Autodesk Fusion 360 part; units mm, degrees
note: some values were not read from the file. Set by a fixed rule: the direction of a hole.
(part 4 of 10)
  line L2847 (66.04, 10.795) -> (64.135, 10.795)
  line L2848 (64.135, 10.795) -> (54.61, 10.795)
  line L2849 (54.61, 10.795) -> (52.07, 10.795)
  line L2850 (67.31, 4.89) -> (67.31, 10.795)
  line L2851 (80.01, 4.89) -> (80.01, 10.795)
  line L2852 (4.635, 10.795) -> (15.24, 10.795)
  line L2853 (15.24, 10.795) -> (15.875, 10.795)
  line L2854 (15.875, 10.795) -> (25.4, 10.795)
  line L2855 (28.575, 10.795) -> (25.4, 10.795)
  line L2856 (28.575, 10.795) -> (38.1, 10.795)
  line L2857 (38.1, 10.795) -> (40.64, 10.795)
  line L2858 (40.64, 10.795) -> (41.275, 10.795)
  line L2859 (41.275, 10.795) -> (52.07, 10.795)
  line L2860 (41.275, 4.89) -> (41.275, 10.795)
  line L2861 (28.575, 4.89) -> (28.575, 10.795)
  line L2862 (15.875, 4.89) -> (15.875, 10.795)
  line L2863 (12.7, 16.51) -> (12.7, 11.43)
  line L2864 (12.7, 11.43) -> (25.4, 11.43)
  line L2865 (25.4, 11.43) -> (25.4, 10.795)
  line L2866 (25.4, 10.795) -> (25.4, 16.51)
  line L2867 (38.1, 16.51) -> (38.1, 10.795)
  line L2868 (64.77, 16.51) -> (64.77, 11.43)
  line L2869 (64.77, 11.43) -> (64.135, 10.795)
  line L2870 (76.2, 16.51) -> (76.2, 10.795)
  line L2871 (87.63, 16.51) -> (87.63, 11.43)
  line L2872 (87.63, 11.43) -> (88.265, 10.795)
  line L2873 (76.2, 76.2) -> (55.245, 76.2)
  line L2874 (55.245, 76.2) -> (54.165, 76.2)
  line L2875 (24.13, 76.835) -> (26.67, 76.835)
  line L2876 (32.8483, 78.7425) -> (32.8508, 78.74)
  line L2877 (50.8, 78.74) -> (32.8508, 78.74)
  line L2878 (26.67, 76.835) -> (28.5775, 78.7425)
  line L2879 (28.5775, 78.7425) -> (32.8483, 78.7425)
  line L2880 (53.34, 75.375) -> (50.8, 77.915)
  line L2881 (50.8, 77.915) -> (50.8, 78.74)
  line L2882 (53.34, 75.375) -> (54.165, 76.2)
  line L2883 (54.165, 76.2) -> (55.245, 76.2)
  line L2884 (88.265, 10.795) -> (95.44, 10.795)
  line L2885 (80.01, 4.89) -> (80.01, 4.445)
  line L2886 (53.34, 75.375) -> (53.34, 60.96)
  line L2887 (53.34, 60.96) -> (50.8, 58.42)
  line L2888 (36.534, 67.1383) -> (37.02, 67.235)
  line L2889 (37.918, 66.863) -> (38.1933, 66.451)
  line L2890 (36.122, 62.527) -> (35.8467, 62.939)
  line L2891 (36.534, 62.2517) -> (36.122, 62.527)
  line L2892 (38.1933, 62.939) -> (37.918, 62.527)
  line L2893 (38.29, 63.425) -> (38.1933, 62.939)
  line L2894 (37.506, 67.1383) -> (37.918, 66.863)
  line L2895 (35.75, 65.965) -> (35.8467, 66.451)
  line L2896 (36.122, 66.863) -> (36.534, 67.1383)
  line L2897 (35.8467, 66.451) -> (36.122, 66.863)
  line L2898 (35.75, 63.425) -> (35.75, 65.965)
  line L2899 (37.506, 62.2517) -> (37.02, 62.155)
  line L2900 (37.02, 62.155) -> (36.534, 62.2517)
  line L2901 (37.918, 62.527) -> (37.506, 62.2517)
  line L2902 (37.02, 67.235) -> (37.506, 67.1383)
  line L2903 (38.29, 65.965) -> (38.29, 63.425)
  line L2904 (38.1933, 66.451) -> (38.29, 65.965)
  line L2905 (35.8467, 62.939) -> (35.75, 63.425)
  line L2906 (2.25, 65.99) -> (2.3467, 66.476)
  line L2907 (3.034, 62.2767) -> (2.622, 62.552)
  line L2908 (4.79, 65.99) -> (4.79, 63.45)
  line L2909 (4.418, 62.552) -> (4.006, 62.2767)
  line L2910 (4.6933, 66.476) -> (4.79, 65.99)
  line L2911 (4.006, 67.1633) -> (4.418, 66.888)
  line L2912 (2.3467, 66.476) -> (2.622, 66.888)
  line L2913 (2.25, 63.45) -> (2.25, 65.99)
  line L2914 (2.3467, 62.964) -> (2.25, 63.45)
  line L2915 (4.79, 63.45) -> (4.6933, 62.964)
  line L2916 (2.622, 62.552) -> (2.3467, 62.964)
  line L2917 (4.006, 62.2767) -> (3.52, 62.18)
  line L2918 (2.622, 66.888) -> (3.034, 67.1633)
  line L2919 (4.6933, 62.964) -> (4.418, 62.552)
  line L2920 (3.034, 67.1633) -> (3.52, 67.26)
  line L2921 (3.52, 67.26) -> (4.006, 67.1633)
  line L2922 (4.418, 66.888) -> (4.6933, 66.476)
  line L2923 (3.52, 62.18) -> (3.034, 62.2767)
  line L2924 (64.208, 67.013) -> (64.4833, 66.601)
  line L2925 (63.31, 62.305) -> (62.824, 62.4017)
  line L2926 (62.412, 62.677) -> (62.1367, 63.089)
  line L2927 (64.4833, 63.089) -> (64.208, 62.677)
  line L2928 (63.796, 62.4017) -> (63.31, 62.305)
  line L2929 (64.208, 62.677) -> (63.796, 62.4017)
  line L2930 (64.58, 66.115) -> (64.58, 63.575)
  line L2931 (64.4833, 66.601) -> (64.58, 66.115)
  line L2932 (64.58, 63.575) -> (64.4833, 63.089)
  line L2933 (62.412, 67.013) -> (62.824, 67.2883)
  line L2934 (63.31, 67.385) -> (63.796, 67.2883)
  line L2935 (62.824, 67.2883) -> (63.31, 67.385)
  line L2936 (63.796, 67.2883) -> (64.208, 67.013)
  line L2937 (62.1367, 66.601) -> (62.412, 67.013)
  line L2938 (62.04, 66.115) -> (62.1367, 66.601)
  line L2939 (62.824, 62.4017) -> (62.412, 62.677)
  line L2940 (62.04, 63.575) -> (62.04, 66.115)
  line L2941 (62.1367, 63.089) -> (62.04, 63.575)
  line L2942 (96.81, 62.28) -> (96.324, 62.3767)
  line L2943 (95.912, 66.988) -> (96.324, 67.2633)
  line L2944 (97.708, 66.988) -> (97.9833, 66.576)
  line L2945 (96.81, 67.36) -> (97.296, 67.2633)
  line L2946 (95.912, 62.652) -> (95.6367, 63.064)
  line L2947 (95.6367, 63.064) -> (95.54, 63.55)
  line L2948 (97.296, 62.3767) -> (96.81, 62.28)
  line L2949 (96.324, 67.2633) -> (96.81, 67.36)
  line L2950 (95.6367, 66.576) -> (95.912, 66.988)
  line L2951 (95.54, 66.09) -> (95.6367, 66.576)
  line L2952 (97.296, 67.2633) -> (97.708, 66.988)
  line L2953 (97.9833, 66.576) -> (98.08, 66.09)
  line L2954 (98.08, 66.09) -> (98.08, 63.55)
  line L2955 (98.08, 63.55) -> (97.9833, 63.064)
  line L2956 (97.9833, 63.064) -> (97.708, 62.652)
  line L2957 (97.708, 62.652) -> (97.296, 62.3767)
  line L2958 (96.324, 62.3767) -> (95.912, 62.652)
  line L2959 (95.54, 63.55) -> (95.54, 66.09)
  line L2960 (8.0863, 54.243) -> (7.811, 53.831)
  line L2961 (3.475, 55.627) -> (3.887, 55.9023)
  line L2962 (6.913, 55.999) -> (7.399, 55.9023)
  line L2963 (8.0863, 55.215) -> (8.183, 54.729)
  line L2964 (3.1997, 54.243) -> (3.103, 54.729)
  line L2965 (4.373, 55.999) -> (6.913, 55.999)
  line L2966 (3.475, 53.831) -> (3.1997, 54.243)
  line L2967 (7.399, 55.9023) -> (7.811, 55.627)
  line L2968 (6.913, 53.459) -> (4.373, 53.459)
  line L2969 (4.373, 53.459) -> (3.887, 53.5557)
  line L2970 (8.183, 54.729) -> (8.0863, 54.243)
  line L2971 (3.103, 54.729) -> (3.1997, 55.215)
  line L2972 (3.887, 53.5557) -> (3.475, 53.831)
  line L2973 (7.811, 55.627) -> (8.0863, 55.215)
  line L2974 (7.811, 53.831) -> (7.399, 53.5557)
  line L2975 (3.887, 55.9023) -> (4.373, 55.999)
  line L2976 (3.1997, 55.215) -> (3.475, 55.627)
  line L2977 (7.399, 53.5557) -> (6.913, 53.459)
  line L2978 (3.887, 30.5557) -> (3.475, 30.831)
  line L2979 (4.373, 30.459) -> (3.887, 30.5557)
  line L2980 (6.913, 30.459) -> (4.373, 30.459)
  line L2981 (7.399, 32.9023) -> (7.811, 32.627)
  line L2982 (8.0863, 32.215) -> (8.183, 31.729)
  line L2983 (7.811, 30.831) -> (7.399, 30.5557)
  line L2984 (4.373, 32.999) -> (6.913, 32.999)
  line L2985 (3.887, 32.9023) -> (4.373, 32.999)
  line L2986 (3.475, 32.627) -> (3.887, 32.9023)
  line L2987 (3.475, 30.831) -> (3.1997, 31.243)
  line L2988 (3.1997, 32.215) -> (3.475, 32.627)
  line L2989 (6.913, 32.999) -> (7.399, 32.9023)
  line L2990 (3.103, 31.729) -> (3.1997, 32.215)
  line L2991 (3.1997, 31.243) -> (3.103, 31.729)
  line L2992 (8.0863, 31.243) -> (7.811, 30.831)
  line L2993 (7.399, 30.5557) -> (6.913, 30.459)
  line L2994 (7.811, 32.627) -> (8.0863, 32.215)
  line L2995 (8.183, 31.729) -> (8.0863, 31.243)
  line L2996 (20.099, 53.5557) -> (19.613, 53.459)
  line L2997 (15.803, 54.729) -> (15.8997, 55.215)
  line L2998 (19.613, 55.999) -> (20.099, 55.9023)
  line L2999 (19.613, 53.459) -> (17.073, 53.459)
  line L3000 (16.587, 53.5557) -> (16.175, 53.831)
  line L3001 (20.7863, 54.243) -> (20.511, 53.831)
  line L3002 (20.7863, 55.215) -> (20.883, 54.729)
  line L3003 (20.511, 55.627) -> (20.7863, 55.215)
  line L3004 (15.8997, 54.243) -> (15.803, 54.729)
  line L3005 (20.511, 53.831) -> (20.099, 53.5557)
  line L3006 (20.883, 54.729) -> (20.7863, 54.243)
  line L3007 (16.175, 53.831) -> (15.8997, 54.243)
  line L3008 (15.8997, 55.215) -> (16.175, 55.627)
  line L3009 (16.175, 55.627) -> (16.587, 55.9023)
  line L3010 (16.587, 55.9023) -> (17.073, 55.999)
  line L3011 (20.099, 55.9023) -> (20.511, 55.627)
  line L3012 (17.073, 53.459) -> (16.587, 53.5557)
  line L3013 (17.073, 55.999) -> (19.613, 55.999)
  line L3014 (15.803, 31.729) -> (15.8997, 32.215)
  line L3015 (17.073, 30.459) -> (16.587, 30.5557)
  line L3016 (20.099, 30.5557) -> (19.613, 30.459)
  line L3017 (15.8997, 31.243) -> (15.803, 31.729)
  line L3018 (16.175, 32.627) -> (16.587, 32.9023)
  line L3019 (16.175, 30.831) -> (15.8997, 31.243)
  line L3020 (16.587, 32.9023) -> (17.073, 32.999)
  line L3021 (20.511, 30.831) -> (20.099, 30.5557)
  line L3022 (20.7863, 31.243) -> (20.511, 30.831)
  line L3023 (19.613, 32.999) -> (20.099, 32.9023)
  line L3024 (20.099, 32.9023) -> (20.511, 32.627)
  line L3025 (17.073, 32.999) -> (19.613, 32.999)
  line L3026 (15.8997, 32.215) -> (16.175, 32.627)
  line L3027 (16.587, 30.5557) -> (16.175, 30.831)
  line L3028 (20.883, 31.729) -> (20.7863, 31.243)
  line L3029 (20.7863, 32.215) -> (20.883, 31.729)
  line L3030 (20.511, 32.627) -> (20.7863, 32.215)
  line L3031 (19.613, 30.459) -> (17.073, 30.459)
  line L3032 (29.287, 53.5557) -> (28.875, 53.831)
  line L3033 (33.583, 54.729) -> (33.4863, 54.243)
  line L3034 (32.313, 55.999) -> (32.799, 55.9023)
  line L3035 (33.211, 53.831) -> (32.799, 53.5557)
  line L3036 (33.4863, 54.243) -> (33.211, 53.831)
  line L3037 (28.875, 53.831) -> (28.5997, 54.243)
  line L3038 (32.799, 55.9023) -> (33.211, 55.627)
  line L3039 (28.5997, 55.215) -> (28.875, 55.627)
  line L3040 (29.773, 53.459) -> (29.287, 53.5557)
  line L3041 (28.875, 55.627) -> (29.287, 55.9023)
  line L3042 (28.503, 54.729) -> (28.5997, 55.215)
  line L3043 (33.4863, 55.215) -> (33.583, 54.729)
  line L3044 (32.799, 53.5557) -> (32.313, 53.459)
  line L3045 (28.5997, 54.243) -> (28.503, 54.729)
  line L3046 (29.287, 55.9023) -> (29.773, 55.999)
  line L3047 (33.211, 55.627) -> (33.4863, 55.215)
  line L3048 (32.313, 53.459) -> (29.773, 53.459)
  line L3049 (29.773, 55.999) -> (32.313, 55.999)
  line L3050 (29.773, 30.459) -> (29.287, 30.5557)
  line L3051 (32.313, 30.459) -> (29.773, 30.459)
  line L3052 (28.875, 30.831) -> (28.5997, 31.243)
  line L3053 (32.799, 30.5557) -> (32.313, 30.459)
  line L3054 (29.287, 30.5557) -> (28.875, 30.831)
  line L3055 (29.287, 32.9023) -> (29.773, 32.999)
  line L3056 (28.875, 32.627) -> (29.287, 32.9023)
  line L3057 (33.211, 32.627) -> (33.4863, 32.215)
  line L3058 (33.583, 31.729) -> (33.4863, 31.243)
  line L3059 (33.4863, 31.243) -> (33.211, 30.831)
  line L3060 (32.799, 32.9023) -> (33.211, 32.627)
  line L3061 (28.5997, 31.243) -> (28.503, 31.729)
  line L3062 (29.773, 32.999) -> (32.313, 32.999)
  line L3063 (28.5997, 32.215) -> (28.875, 32.627)
  line L3064 (33.211, 30.831) -> (32.799, 30.5557)
  line L3065 (33.4863, 32.215) -> (33.583, 31.729)
  line L3066 (32.313, 32.999) -> (32.799, 32.9023)
  line L3067 (28.503, 31.729) -> (28.5997, 32.215)
  line L3068 (41.575, 55.627) -> (41.987, 55.9023)
  line L3069 (45.499, 53.5557) -> (45.013, 53.459)
  line L3070 (41.987, 53.5557) -> (41.575, 53.831)
  line L3071 (45.499, 55.9023) -> (45.911, 55.627)
  line L3072 (41.575, 53.831) -> (41.2997, 54.243)
  line L3073 (46.283, 54.729) -> (46.1863, 54.243)
  line L3074 (41.2997, 54.243) -> (41.203, 54.729)
  line L3075 (45.911, 53.831) -> (45.499, 53.5557)
  line L3076 (45.013, 53.459) -> (42.473, 53.459)
  line L3077 (42.473, 55.999) -> (45.013, 55.999)
  line L3078 (45.013, 55.999) -> (45.499, 55.9023)
  line L3079 (41.203, 54.729) -> (41.2997, 55.215)
  line L3080 (46.1863, 55.215) -> (46.283, 54.729)
  line L3081 (45.911, 55.627) -> (46.1863, 55.215)
  line L3082 (41.987, 55.9023) -> (42.473, 55.999)
  line L3083 (41.2997, 55.215) -> (41.575, 55.627)
  line L3084 (42.473, 53.459) -> (41.987, 53.5557)
  line L3085 (46.1863, 54.243) -> (45.911, 53.831)
  line L3086 (45.911, 30.831) -> (45.499, 30.5557)
  line L3087 (46.1863, 32.215) -> (46.283, 31.729)
  line L3088 (45.013, 32.999) -> (45.499, 32.9023)
  line L3089 (45.911, 32.627) -> (46.1863, 32.215)
  line L3090 (46.1863, 31.243) -> (45.911, 30.831)
  line L3091 (45.499, 32.9023) -> (45.911, 32.627)
  line L3092 (45.013, 30.459) -> (42.473, 30.459)
  line L3093 (41.203, 31.729) -> (41.2997, 32.215)
  line L3094 (41.2997, 31.243) -> (41.203, 31.729)
  line L3095 (42.473, 30.459) -> (41.987, 30.5557)
  line L3096 (46.283, 31.729) -> (46.1863, 31.243)
  line L3097 (41.575, 32.627) -> (41.987, 32.9023)
  line L3098 (42.473, 32.999) -> (45.013, 32.999)
  line L3099 (41.987, 32.9023) -> (42.473, 32.999)
  line L3100 (41.575, 30.831) -> (41.2997, 31.243)
  line L3101 (41.2997, 32.215) -> (41.575, 32.627)
  line L3102 (41.987, 30.5557) -> (41.575, 30.831)
  line L3103 (45.499, 30.5557) -> (45.013, 30.459)
  line L3104 (58.348, 55.999) -> (58.834, 55.9023)
  line L3105 (55.808, 55.999) -> (58.348, 55.999)
  line L3106 (54.91, 55.627) -> (55.322, 55.9023)
  line L3107 (54.6347, 54.243) -> (54.538, 54.729)
  line L3108 (58.834, 53.5557) -> (58.348, 53.459)
  line L3109 (55.322, 53.5557) -> (54.91, 53.831)
  line L3110 (59.5213, 55.215) -> (59.618, 54.729)
  line L3111 (58.834, 55.9023) -> (59.246, 55.627)
  line L3112 (54.6347, 55.215) -> (54.91, 55.627)
  line L3113 (55.808, 53.459) -> (55.322, 53.5557)
  line L3114 (59.246, 53.831) -> (58.834, 53.5557)
  line L3115 (58.348, 53.459) -> (55.808, 53.459)
  line L3116 (59.618, 54.729) -> (59.5213, 54.243)
  line L3117 (59.5213, 54.243) -> (59.246, 53.831)
  line L3118 (59.246, 55.627) -> (59.5213, 55.215)
  line L3119 (54.538, 54.729) -> (54.6347, 55.215)
  line L3120 (55.322, 55.9023) -> (55.808, 55.999)
  line L3121 (54.91, 53.831) -> (54.6347, 54.243)
  line L3122 (54.6347, 31.243) -> (54.538, 31.729)
  line L3123 (59.618, 31.729) -> (59.5213, 31.243)
  line L3124 (59.246, 32.627) -> (59.5213, 32.215)
  line L3125 (54.6347, 32.215) -> (54.91, 32.627)
  line L3126 (59.5213, 32.215) -> (59.618, 31.729)
  line L3127 (59.5213, 31.243) -> (59.246, 30.831)
  line L3128 (54.91, 30.831) -> (54.6347, 31.243)
  line L3129 (55.808, 30.459) -> (55.322, 30.5557)
  line L3130 (58.348, 30.459) -> (55.808, 30.459)
  line L3131 (55.322, 32.9023) -> (55.808, 32.999)
  line L3132 (58.834, 32.9023) -> (59.246, 32.627)
  line L3133 (59.246, 30.831) -> (58.834, 30.5557)
  line L3134 (54.538, 31.729) -> (54.6347, 32.215)
  line L3135 (55.808, 32.999) -> (58.348, 32.999)
  line L3136 (54.91, 32.627) -> (55.322, 32.9023)
  line L3137 (58.348, 32.999) -> (58.834, 32.9023)
  line L3138 (58.834, 30.5557) -> (58.348, 30.459)
  line L3139 (55.322, 30.5557) -> (54.91, 30.831)
  line L3140 (72.318, 54.729) -> (72.2213, 54.243)
  line L3141 (68.022, 55.9023) -> (68.508, 55.999)
  line L3142 (71.534, 55.9023) -> (71.946, 55.627)
  line L3143 (67.3347, 55.215) -> (67.61, 55.627)
  line L3144 (71.946, 53.831) -> (71.534, 53.5557)
  line L3145 (68.508, 55.999) -> (71.048, 55.999)
  line L3146 (72.2213, 55.215) -> (72.318, 54.729)
  line L3147 (67.61, 55.627) -> (68.022, 55.9023)
  line L3148 (67.61, 53.831) -> (67.3347, 54.243)
  line L3149 (72.2213, 54.243) -> (71.946, 53.831)
  line L3150 (68.508, 53.459) -> (68.022, 53.5557)
  line L3151 (67.238, 54.729) -> (67.3347, 55.215)
  line L3152 (71.534, 53.5557) -> (71.048, 53.459)
  line L3153 (71.048, 55.999) -> (71.534, 55.9023)
  line L3154 (67.3347, 54.243) -> (67.238, 54.729)
  line L3155 (68.022, 53.5557) -> (67.61, 53.831)
  line L3156 (71.946, 55.627) -> (72.2213, 55.215)
  line L3157 (71.048, 53.459) -> (68.508, 53.459)
  line L3158 (68.508, 30.459) -> (68.022, 30.5557)
  line L3159 (68.022, 30.5557) -> (67.61, 30.831)
  line L3160 (71.946, 32.627) -> (72.2213, 32.215)
  line L3161 (71.946, 30.831) -> (71.534, 30.5557)
  line L3162 (72.2213, 31.243) -> (71.946, 30.831)
  line L3163 (71.048, 30.459) -> (68.508, 30.459)
  line L3164 (67.238, 31.729) -> (67.3347, 32.215)
  line L3165 (67.3347, 32.215) -> (67.61, 32.627)
  line L3166 (72.2213, 32.215) -> (72.318, 31.729)
  line L3167 (71.534, 32.9023) -> (71.946, 32.627)
  line L3168 (71.048, 32.999) -> (71.534, 32.9023)
  line L3169 (68.508, 32.999) -> (71.048, 32.999)
  line L3170 (67.61, 32.627) -> (68.022, 32.9023)
  line L3171 (67.61, 30.831) -> (67.3347, 31.243)
  line L3172 (68.022, 32.9023) -> (68.508, 32.999)
  line L3173 (67.3347, 31.243) -> (67.238, 31.729)
  line L3174 (72.318, 31.729) -> (72.2213, 31.243)
  line L3175 (71.534, 30.5557) -> (71.048, 30.459)
  line L3176 (84.9213, 54.243) -> (84.646, 53.831)
  line L3177 (80.722, 53.5557) -> (80.31, 53.831)
  line L3178 (80.0347, 54.243) -> (79.938, 54.729)
  line L3179 (81.208, 55.999) -> (83.748, 55.999)
  line L3180 (79.938, 54.729) -> (80.0347, 55.215)
  line L3181 (83.748, 53.459) -> (81.208, 53.459)
  line L3182 (84.9213, 55.215) -> (85.018, 54.729)
  line L3183 (81.208, 53.459) -> (80.722, 53.5557)
  line L3184 (83.748, 55.999) -> (84.234, 55.9023)
  line L3185 (84.646, 55.627) -> (84.9213, 55.215)
  line L3186 (80.31, 53.831) -> (80.0347, 54.243)
  line L3187 (84.646, 53.831) -> (84.234, 53.5557)
  line L3188 (84.234, 55.9023) -> (84.646, 55.627)
  line L3189 (85.018, 54.729) -> (84.9213, 54.243)
  line L3190 (80.722, 55.9023) -> (81.208, 55.999)
  line L3191 (84.234, 53.5557) -> (83.748, 53.459)
  line L3192 (80.31, 55.627) -> (80.722, 55.9023)
  line L3193 (80.0347, 55.215) -> (80.31, 55.627)
  line L3194 (84.9213, 32.215) -> (85.018, 31.729)
  line L3195 (83.748, 30.459) -> (81.208, 30.459)
  line L3196 (83.748, 32.999) -> (84.234, 32.9023)
  line L3197 (84.234, 32.9023) -> (84.646, 32.627)
  line L3198 (79.938, 31.729) -> (80.0347, 32.215)
  line L3199 (84.234, 30.5557) -> (83.748, 30.459)
  line L3200 (80.0347, 32.215) -> (80.31, 32.627)
  line L3201 (81.208, 32.999) -> (83.748, 32.999)
  line L3202 (81.208, 30.459) -> (80.722, 30.5557)
  line L3203 (84.646, 32.627) -> (84.9213, 32.215)
  line L3204 (80.31, 32.627) -> (80.722, 32.9023)
  line L3205 (85.018, 31.729) -> (84.9213, 31.243)
  line L3206 (80.0347, 31.243) -> (79.938, 31.729)
  line L3207 (84.9213, 31.243) -> (84.646, 30.831)
  line L3208 (80.31, 30.831) -> (80.0347, 31.243)
  line L3209 (80.722, 32.9023) -> (81.208, 32.999)
  line L3210 (80.722, 30.5557) -> (80.31, 30.831)
  line L3211 (84.646, 30.831) -> (84.234, 30.5557)
  line L3212 (95.813, 55.999) -> (96.299, 55.9023)
  line L3213 (93.273, 55.999) -> (95.813, 55.999)
  line L3214 (96.711, 55.627) -> (96.9863, 55.215)
  line L3215 (92.003, 54.729) -> (92.0997, 55.215)
  line L3216 (95.813, 53.459) -> (93.273, 53.459)
  line L3217 (92.375, 53.831) -> (92.0997, 54.243)
  line L3218 (92.375, 55.627) -> (92.787, 55.9023)
  line L3219 (96.711, 53.831) -> (96.299, 53.5557)
  line L3220 (96.9863, 55.215) -> (97.083, 54.729)
  line L3221 (96.299, 53.5557) -> (95.813, 53.459)
  line L3222 (92.0997, 54.243) -> (92.003, 54.729)
  line L3223 (92.0997, 55.215) -> (92.375, 55.627)
  line L3224 (93.273, 53.459) -> (92.787, 53.5557)
  line L3225 (96.299, 55.9023) -> (96.711, 55.627)
  line L3226 (96.9863, 54.243) -> (96.711, 53.831)
  line L3227 (97.083, 54.729) -> (96.9863, 54.243)
  line L3228 (92.787, 53.5557) -> (92.375, 53.831)
  line L3229 (92.787, 55.9023) -> (93.273, 55.999)
  line L3230 (93.273, 30.459) -> (92.787, 30.5557)
  line L3231 (96.299, 32.9023) -> (96.711, 32.627)
  line L3232 (95.813, 32.999) -> (96.299, 32.9023)
  line L3233 (96.9863, 32.215) -> (97.083, 31.729)
  line L3234 (96.9863, 31.243) -> (96.711, 30.831)
  line L3235 (96.711, 30.831) -> (96.299, 30.5557)
  line L3236 (92.375, 30.831) -> (92.0997, 31.243)
  line L3237 (97.083, 31.729) -> (96.9863, 31.243)
  line L3238 (92.787, 32.9023) -> (93.273, 32.999)
  line L3239 (92.375, 32.627) -> (92.787, 32.9023)
  line L3240 (93.273, 32.999) -> (95.813, 32.999)
  line L3241 (92.003, 31.729) -> (92.0997, 32.215)
  line L3242 (92.0997, 32.215) -> (92.375, 32.627)
  line L3243 (96.299, 30.5557) -> (95.813, 30.459)
  line L3244 (95.813, 30.459) -> (93.273, 30.459)
  line L3245 (92.0997, 31.243) -> (92.003, 31.729)
  line L3246 (92.787, 30.5557) -> (92.375, 30.831)
  line L3247 (96.711, 32.627) -> (96.9863, 32.215)
  line L3248 (48.26, 77.475) -> (48.6618, 77.3951)
  line L3249 (47.5175, 73.5825) -> (47.2899, 73.9232)
  line L3250 (47.21, 74.325) -> (47.21, 76.425)
  line L3251 (48.6618, 77.3951) -> (49.0025, 77.1675)
  line L3252 (49.0025, 73.5825) -> (48.6618, 73.3549)
  line L3253 (49.31, 74.325) -> (49.2301, 73.9232)
  line L3254 (47.21, 76.425) -> (47.2899, 76.8268)
  line L3255 (49.31, 76.425) -> (49.31, 74.325)
  line L3256 (49.0025, 77.1675) -> (49.2301, 76.8268)
  line L3257 (47.5175, 77.1675) -> (47.8582, 77.3951)
  line L3258 (47.8582, 73.3549) -> (47.5175, 73.5825)
  line L3259 (49.2301, 76.8268) -> (49.31, 76.425)
  line L3260 (49.2301, 73.9232) -> (49.0025, 73.5825)
  line L3261 (47.2899, 76.8268) -> (47.5175, 77.1675)
  line L3262 (47.8582, 77.3951) -> (48.26, 77.475)
  line L3263 (47.2899, 73.9232) -> (47.21, 74.325)
  line L3264 (48.26, 73.275) -> (47.8582, 73.3549)
  line L3265 (48.6618, 73.3549) -> (48.26, 73.275)
  line L3266 (52.3699, 76.8268) -> (52.5975, 77.1675)
  line L3267 (54.3101, 76.8268) -> (54.39, 76.425)
  line L3268 (52.5975, 73.5825) -> (52.3699, 73.9232)
  line L3269 (52.29, 74.325) -> (52.29, 76.425)
  line L3270 (52.3699, 73.9232) -> (52.29, 74.325)
  line L3271 (52.9382, 77.3951) -> (53.34, 77.475)
  line L3272 (53.7418, 77.3951) -> (54.0825, 77.1675)
  line L3273 (54.3101, 73.9232) -> (54.0825, 73.5825)
  line L3274 (54.0825, 77.1675) -> (54.3101, 76.8268)
  line L3275 (52.29, 76.425) -> (52.3699, 76.8268)
  line L3276 (52.5975, 77.1675) -> (52.9382, 77.3951)
  line L3277 (53.7418, 73.3549) -> (53.34, 73.275)
  line L3278 (53.34, 73.275) -> (52.9382, 73.3549)
  line L3279 (54.39, 76.425) -> (54.39, 74.325)
  line L3280 (54.39, 74.325) -> (54.3101, 73.9232)
  line L3281 (53.34, 77.475) -> (53.7418, 77.3951)
  line L3282 (54.0825, 73.5825) -> (53.7418, 73.3549)
  line L3283 (52.9382, 73.3549) -> (52.5975, 73.5825)
  line L3284 (2.535, 10.795) -> (2.6149, 11.1968)
  line L3285 (6.4275, 10.0525) -> (6.0868, 9.8249)
  line L3286 (6.6551, 11.1968) -> (6.735, 10.795)
  line L3287 (5.685, 9.745) -> (3.585, 9.745)
  line L3288 (3.1832, 11.7651) -> (3.585, 11.845)
  line L3289 (3.1832, 9.8249) -> (2.8425, 10.0525)
  line L3290 (6.4275, 11.5375) -> (6.6551, 11.1968)
  line L3291 (6.6551, 10.3932) -> (6.4275, 10.0525)
  line L3292 (2.6149, 11.1968) -> (2.8425, 11.5375)
  line L3293 (6.735, 10.795) -> (6.6551, 10.3932)
  line L3294 (3.585, 9.745) -> (3.1832, 9.8249)
  line L3295 (2.6149, 10.3932) -> (2.535, 10.795)
  line L3296 (2.8425, 11.5375) -> (3.1832, 11.7651)
  line L3297 (2.8425, 10.0525) -> (2.6149, 10.3932)
  line L3298 (6.0868, 9.8249) -> (5.685, 9.745)
  line L3299 (5.685, 11.845) -> (6.0868, 11.7651)
  line L3300 (6.0868, 11.7651) -> (6.4275, 11.5375)
  line L3301 (3.585, 11.845) -> (5.685, 11.845)
  line L3302 (6.6551, 15.4732) -> (6.4275, 15.1325)
  line L3303 (5.685, 14.825) -> (3.585, 14.825)
  line L3304 (6.0868, 14.9049) -> (5.685, 14.825)
  line L3305 (6.6551, 16.2768) -> (6.735, 15.875)
  line L3306 (3.585, 16.925) -> (5.685, 16.925)
  line L3307 (2.535, 15.875) -> (2.6149, 16.2768)
  line L3308 (2.8425, 16.6175) -> (3.1832, 16.8451)
  line L3309 (2.6149, 15.4732) -> (2.535, 15.875)
  line L3310 (2.8425, 15.1325) -> (2.6149, 15.4732)
  line L3311 (6.735, 15.875) -> (6.6551, 15.4732)
  line L3312 (3.1832, 16.8451) -> (3.585, 16.925)
  line L3313 (6.4275, 16.6175) -> (6.6551, 16.2768)
  line L3314 (6.0868, 16.8451) -> (6.4275, 16.6175)
  line L3315 (3.1832, 14.9049) -> (2.8425, 15.1325)
  line L3316 (2.6149, 16.2768) -> (2.8425, 16.6175)
  line L3317 (3.585, 14.825) -> (3.1832, 14.9049)
  line L3318 (6.4275, 15.1325) -> (6.0868, 14.9049)
  line L3319 (5.685, 16.925) -> (6.0868, 16.8451)
  line L3320 (16.6175, 3.0975) -> (16.2768, 2.8699)
  line L3321 (16.6175, 6.6825) -> (16.8451, 6.3418)
  line L3322 (16.2768, 6.9101) -> (16.6175, 6.6825)
  line L3323 (15.875, 2.79) -> (15.4732, 2.8699)
  line L3324 (14.9049, 6.3418) -> (15.1325, 6.6825)
  line L3325 (16.925, 3.84) -> (16.8451, 3.4382)
  line L3326 (14.825, 5.94) -> (14.9049, 6.3418)
  line L3327 (15.1325, 3.0975) -> (14.9049, 3.4382)
  line L3328 (15.4732, 2.8699) -> (15.1325, 3.0975)
  line L3329 (14.9049, 3.4382) -> (14.825, 3.84)
  line L3330 (14.825, 3.84) -> (14.825, 5.94)
  line L3331 (16.925, 5.94) -> (16.925, 3.84)
  line L3332 (15.875, 6.99) -> (16.2768, 6.9101)
  line L3333 (16.2768, 2.8699) -> (15.875, 2.79)
  line L3334 (15.1325, 6.6825) -> (15.4732, 6.9101)
  line L3335 (16.8451, 3.4382) -> (16.6175, 3.0975)
  line L3336 (15.4732, 6.9101) -> (15.875, 6.99)
  line L3337 (16.8451, 6.3418) -> (16.925, 5.94)
  line L3338 (19.905, 5.94) -> (19.9849, 6.3418)
  line L3339 (21.6975, 6.6825) -> (21.9251, 6.3418)
  line L3340 (21.9251, 3.4382) -> (21.6975, 3.0975)
  line L3341 (22.005, 5.94) -> (22.005, 3.84)
  line L3342 (20.955, 6.99) -> (21.3568, 6.9101)
  line L3343 (20.2125, 6.6825) -> (20.5532, 6.9101)
  line L3344 (19.9849, 3.4382) -> (19.905, 3.84)
  line L3345 (20.955, 2.79) -> (20.5532, 2.8699)
  line L3346 (20.2125, 3.0975) -> (19.9849, 3.4382)
  line L3347 (19.9849, 6.3418) -> (20.2125, 6.6825)
  line L3348 (21.9251, 6.3418) -> (22.005, 5.94)
  line L3349 (20.5532, 2.8699) -> (20.2125, 3.0975)
  line L3350 (21.3568, 2.8699) -> (20.955, 2.79)
  line L3351 (21.3568, 6.9101) -> (21.6975, 6.6825)
  line L3352 (22.005, 3.84) -> (21.9251, 3.4382)
  line L3353 (21.6975, 3.0975) -> (21.3568, 2.8699)
  line L3354 (19.905, 3.84) -> (19.905, 5.94)
  line L3355 (20.5532, 6.9101) -> (20.955, 6.99)
  line L3356 (28.9768, 2.8699) -> (28.575, 2.79)
  line L3357 (27.525, 3.84) -> (27.525, 5.94)
  line L3358 (29.3175, 6.6825) -> (29.5451, 6.3418)
  line L3359 (27.6049, 6.3418) -> (27.8325, 6.6825)
  line L3360 (27.8325, 6.6825) -> (28.1732, 6.9101)
  line L3361 (29.625, 3.84) -> (29.5451, 3.4382)
  line L3362 (29.5451, 6.3418) -> (29.625, 5.94)
  line L3363 (29.625, 5.94) -> (29.625, 3.84)
  line L3364 (27.525, 5.94) -> (27.6049, 6.3418)
  line L3365 (28.9768, 6.9101) -> (29.3175, 6.6825)
  line L3366 (28.575, 2.79) -> (28.1732, 2.8699)
  line L3367 (29.3175, 3.0975) -> (28.9768, 2.8699)
  line L3368 (28.1732, 6.9101) -> (28.575, 6.99)
  line L3369 (28.1732, 2.8699) -> (27.8325, 3.0975)
  line L3370 (29.5451, 3.4382) -> (29.3175, 3.0975)
  line L3371 (27.8325, 3.0975) -> (27.6049, 3.4382)
  line L3372 (28.575, 6.99) -> (28.9768, 6.9101)
  line L3373 (27.6049, 3.4382) -> (27.525, 3.84)
  line L3374 (34.0568, 6.9101) -> (34.3975, 6.6825)
  line L3375 (34.6251, 3.4382) -> (34.3975, 3.0975)
  line L3376 (34.705, 5.94) -> (34.705, 3.84)
  line L3377 (34.705, 3.84) -> (34.6251, 3.4382)
  line L3378 (34.3975, 3.0975) -> (34.0568, 2.8699)
  line L3379 (34.6251, 6.3418) -> (34.705, 5.94)
  line L3380 (32.9125, 3.0975) -> (32.6849, 3.4382)
  line L3381 (32.6849, 3.4382) -> (32.605, 3.84)
  line L3382 (33.2532, 2.8699) -> (32.9125, 3.0975)
  line L3383 (34.0568, 2.8699) -> (33.655, 2.79)
  line L3384 (34.3975, 6.6825) -> (34.6251, 6.3418)
  line L3385 (32.605, 5.94) -> (32.6849, 6.3418)
  line L3386 (33.2532, 6.9101) -> (33.655, 6.99)
  line L3387 (33.655, 2.79) -> (33.2532, 2.8699)
  line L3388 (32.6849, 6.3418) -> (32.9125, 6.6825)
  line L3389 (33.655, 6.99) -> (34.0568, 6.9101)
  line L3390 (32.605, 3.84) -> (32.605, 5.94)
  line L3391 (32.9125, 6.6825) -> (33.2532, 6.9101)
  line L3392 (41.6768, 2.8699) -> (41.275, 2.79)
  line L3393 (40.5325, 6.6825) -> (40.8732, 6.9101)
  line L3394 (42.2451, 3.4382) -> (42.0175, 3.0975)
  line L3395 (40.225, 5.94) -> (40.3049, 6.3418)
  line L3396 (42.325, 5.94) -> (42.325, 3.84)
  line L3397 (41.6768, 6.9101) -> (42.0175, 6.6825)
  line L3398 (40.8732, 2.8699) -> (40.5325, 3.0975)
  line L3399 (40.5325, 3.0975) -> (40.3049, 3.4382)
  line L3400 (40.8732, 6.9101) -> (41.275, 6.99)
  line L3401 (41.275, 6.99) -> (41.6768, 6.9101)
  line L3402 (40.225, 3.84) -> (40.225, 5.94)
  line L3403 (42.325, 3.84) -> (42.2451, 3.4382)
  line L3404 (40.3049, 6.3418) -> (40.5325, 6.6825)
  line L3405 (40.3049, 3.4382) -> (40.225, 3.84)
  line L3406 (42.0175, 3.0975) -> (41.6768, 2.8699)
  line L3407 (42.0175, 6.6825) -> (42.2451, 6.3418)
  line L3408 (41.275, 2.79) -> (40.8732, 2.8699)
  line L3409 (42.2451, 6.3418) -> (42.325, 5.94)
  line L3410 (45.9532, 2.8699) -> (45.6125, 3.0975)
  line L3411 (46.355, 2.79) -> (45.9532, 2.8699)
  line L3412 (45.3849, 3.4382) -> (45.305, 3.84)
  line L3413 (45.9532, 6.9101) -> (46.355, 6.99)
  line L3414 (45.305, 5.94) -> (45.3849, 6.3418)
  line L3415 (46.355, 6.99) -> (46.7568, 6.9101)
  line L3416 (47.405, 3.84) -> (47.3251, 3.4382)
  line L3417 (47.3251, 3.4382) -> (47.0975, 3.0975)
  line L3418 (47.405, 5.94) -> (47.405, 3.84)
  line L3419 (46.7568, 2.8699) -> (46.355, 2.79)
  line L3420 (45.3849, 6.3418) -> (45.6125, 6.6825)
  line L3421 (45.305, 3.84) -> (45.305, 5.94)
  line L3422 (47.3251, 6.3418) -> (47.405, 5.94)
  line L3423 (47.0975, 6.6825) -> (47.3251, 6.3418)
  line L3424 (45.6125, 3.0975) -> (45.3849, 3.4382)
  line L3425 (46.7568, 6.9101) -> (47.0975, 6.6825)
  line L3426 (45.6125, 6.6825) -> (45.9532, 6.9101)
  line L3427 (47.0975, 3.0975) -> (46.7568, 2.8699)
  line L3428 (55.66, 3.84) -> (55.5801, 3.4382)
  line L3429 (54.61, 6.99) -> (55.0118, 6.9101)
  line L3430 (55.0118, 2.8699) -> (54.61, 2.79)
  line L3431 (55.3525, 3.0975) -> (55.0118, 2.8699)
  line L3432 (55.66, 5.94) -> (55.66, 3.84)
  line L3433 (53.56, 3.84) -> (53.56, 5.94)
  line L3434 (53.8675, 3.0975) -> (53.6399, 3.4382)
  line L3435 (55.5801, 3.4382) -> (55.3525, 3.0975)
  line L3436 (54.2082, 2.8699) -> (53.8675, 3.0975)
  line L3437 (55.5801, 6.3418) -> (55.66, 5.94)
  line L3438 (53.6399, 3.4382) -> (53.56, 3.84)
  line L3439 (54.2082, 6.9101) -> (54.61, 6.99)
  line L3440 (53.8675, 6.6825) -> (54.2082, 6.9101)
  line L3441 (55.0118, 6.9101) -> (55.3525, 6.6825)
  line L3442 (55.3525, 6.6825) -> (55.5801, 6.3418)
  line L3443 (53.6399, 6.3418) -> (53.8675, 6.6825)
  line L3444 (54.61, 2.79) -> (54.2082, 2.8699)
  line L3445 (53.56, 5.94) -> (53.6399, 6.3418)
  line L3446 (58.7199, 3.4382) -> (58.64, 3.84)
  line L3447 (60.0918, 6.9101) -> (60.4325, 6.6825)
  line L3448 (59.2882, 6.9101) -> (59.69, 6.99)
  line L3449 (58.7199, 6.3418) -> (58.9475, 6.6825)
  line L3450 (60.0918, 2.8699) -> (59.69, 2.79)
  line L3451 (58.64, 3.84) -> (58.64, 5.94)
  line L3452 (59.69, 6.99) -> (60.0918, 6.9101)
  line L3453 (58.9475, 3.0975) -> (58.7199, 3.4382)
  line L3454 (60.4325, 3.0975) -> (60.0918, 2.8699)
  line L3455 (60.6601, 3.4382) -> (60.4325, 3.0975)
  line L3456 (58.64, 5.94) -> (58.7199, 6.3418)
  line L3457 (59.2882, 2.8699) -> (58.9475, 3.0975)
  line L3458 (60.4325, 6.6825) -> (60.6601, 6.3418)
  line L3459 (60.6601, 6.3418) -> (60.74, 5.94)
  line L3460 (60.74, 5.94) -> (60.74, 3.84)
  line L3461 (58.9475, 6.6825) -> (59.2882, 6.9101)
  line L3462 (60.74, 3.84) -> (60.6601, 3.4382)
  line L3463 (59.69, 2.79) -> (59.2882, 2.8699)
  line L3464 (68.0525, 6.6825) -> (68.2801, 6.3418)
  line L3465 (66.3399, 3.4382) -> (66.26, 3.84)
  line L3466 (66.26, 5.94) -> (66.3399, 6.3418)
  line L3467 (66.3399, 6.3418) -> (66.5675, 6.6825)
  line L3468 (67.7118, 2.8699) -> (67.31, 2.79)
  line L3469 (66.5675, 3.0975) -> (66.3399, 3.4382)
  line L3470 (67.31, 2.79) -> (66.9082, 2.8699)
  line L3471 (66.26, 3.84) -> (66.26, 5.94)
  line L3472 (67.31, 6.99) -> (67.7118, 6.9101)
  line L3473 (66.9082, 2.8699) -> (66.5675, 3.0975)
  line L3474 (66.5675, 6.6825) -> (66.9082, 6.9101)
  line L3475 (66.9082, 6.9101) -> (67.31, 6.99)
  line L3476 (68.36, 3.84) -> (68.2801, 3.4382)
  line L3477 (68.2801, 3.4382) -> (68.0525, 3.0975)
  line L3478 (68.2801, 6.3418) -> (68.36, 5.94)
  line L3479 (67.7118, 6.9101) -> (68.0525, 6.6825)
  line L3480 (68.0525, 3.0975) -> (67.7118, 2.8699)
  line L3481 (68.36, 5.94) -> (68.36, 3.84)
  line L3482 (73.3601, 3.4382) -> (73.1325, 3.0975)
  line L3483 (71.34, 5.94) -> (71.4199, 6.3418)
  line L3484 (73.44, 3.84) -> (73.3601, 3.4382)
  line L3485 (72.7918, 6.9101) -> (73.1325, 6.6825)
  line L3486 (71.9882, 6.9101) -> (72.39, 6.99)
  line L3487 (73.1325, 6.6825) -> (73.3601, 6.3418)
  line L3488 (71.6475, 6.6825) -> (71.9882, 6.9101)
  line L3489 (71.34, 3.84) -> (71.34, 5.94)
  line L3490 (71.9882, 2.8699) -> (71.6475, 3.0975)
  line L3491 (72.39, 2.79) -> (71.9882, 2.8699)
  line L3492 (71.4199, 3.4382) -> (71.34, 3.84)
  line L3493 (72.7918, 2.8699) -> (72.39, 2.79)
  line L3494 (73.44, 5.94) -> (73.44, 3.84)
  line L3495 (73.1325, 3.0975) -> (72.7918, 2.8699)
  line L3496 (72.39, 6.99) -> (72.7918, 6.9101)
  line L3497 (71.4199, 6.3418) -> (71.6475, 6.6825)
  line L3498 (71.6475, 3.0975) -> (71.4199, 3.4382)
  line L3499 (73.3601, 6.3418) -> (73.44, 5.94)
  line L3500 (81.06, 5.94) -> (81.06, 3.84)
  line L3501 (80.9801, 3.4382) -> (80.7525, 3.0975)
  line L3502 (79.2675, 3.0975) -> (79.0399, 3.4382)
  line L3503 (78.96, 3.84) -> (78.96, 5.94)
  line L3504 (79.6082, 6.9101) -> (80.01, 6.99)
  line L3505 (80.7525, 6.6825) -> (80.9801, 6.3418)
  line L3506 (80.4118, 2.8699) -> (80.01, 2.79)
  line L3507 (80.9801, 6.3418) -> (81.06, 5.94)
  line L3508 (78.96, 5.94) -> (79.0399, 6.3418)
  line L3509 (80.01, 6.99) -> (80.4118, 6.9101)
  line L3510 (79.0399, 3.4382) -> (78.96, 3.84)
  line L3511 (79.0399, 6.3418) -> (79.2675, 6.6825)
  line L3512 (80.01, 2.79) -> (79.6082, 2.8699)
  line L3513 (80.7525, 3.0975) -> (80.4118, 2.8699)
  line L3514 (81.06, 3.84) -> (80.9801, 3.4382)
  line L3515 (79.6082, 2.8699) -> (79.2675, 3.0975)
  line L3516 (80.4118, 6.9101) -> (80.7525, 6.6825)
  line L3517 (79.2675, 6.6825) -> (79.6082, 6.9101)
  line L3518 (84.3475, 3.0975) -> (84.1199, 3.4382)
  line L3519 (85.4918, 6.9101) -> (85.8325, 6.6825)
  line L3520 (85.09, 2.79) -> (84.6882, 2.8699)
  line L3521 (85.8325, 6.6825) -> (86.0601, 6.3418)
  line L3522 (84.04, 3.84) -> (84.04, 5.94)
  line L3523 (84.6882, 2.8699) -> (84.3475, 3.0975)
  line L3524 (86.14, 3.84) -> (86.0601, 3.4382)
  line L3525 (84.1199, 3.4382) -> (84.04, 3.84)
  line L3526 (86.0601, 6.3418) -> (86.14, 5.94)
  line L3527 (85.4918, 2.8699) -> (85.09, 2.79)
  line L3528 (84.1199, 6.3418) -> (84.3475, 6.6825)
  line L3529 (85.8325, 3.0975) -> (85.4918, 2.8699)
  line L3530 (84.04, 5.94) -> (84.1199, 6.3418)
  line L3531 (84.3475, 6.6825) -> (84.6882, 6.9101)
  line L3532 (85.09, 6.99) -> (85.4918, 6.9101)
  line L3533 (84.6882, 6.9101) -> (85.09, 6.99)
  line L3534 (86.14, 5.94) -> (86.14, 3.84)
  line L3535 (86.0601, 3.4382) -> (85.8325, 3.0975)
  line L3536 (96.49, 9.745) -> (94.39, 9.745)
  line L3537 (93.6475, 11.5375) -> (93.9882, 11.7651)
  line L3538 (97.4601, 10.3932) -> (97.2325, 10.0525)
  line L3539 (97.2325, 11.5375) -> (97.4601, 11.1968)
  line L3540 (97.4601, 11.1968) -> (97.54, 10.795)
  line L3541 (93.6475, 10.0525) -> (93.4199, 10.3932)
  line L3542 (93.34, 10.795) -> (93.4199, 11.1968)
  line L3543 (94.39, 9.745) -> (93.9882, 9.8249)
  line L3544 (96.49, 11.845) -> (96.8918, 11.7651)
  line L3545 (97.2325, 10.0525) -> (96.8918, 9.8249)
  line L3546 (93.9882, 9.8249) -> (93.6475, 10.0525)
  line L3547 (96.8918, 9.8249) -> (96.49, 9.745)
  line L3548 (93.4199, 10.3932) -> (93.34, 10.795)
  line L3549 (94.39, 11.845) -> (96.49, 11.845)
  line L3550 (96.8918, 11.7651) -> (97.2325, 11.5375)
  line L3551 (97.54, 10.795) -> (97.4601, 10.3932)
  line L3552 (93.4199, 11.1968) -> (93.6475, 11.5375)
  line L3553 (93.9882, 11.7651) -> (94.39, 11.845)
  line L3554 (93.34, 15.875) -> (93.4199, 16.2768)
  line L3555 (96.8918, 14.9049) -> (96.49, 14.825)
  line L3556 (93.9882, 14.9049) -> (93.6475, 15.1325)
  line L3557 (96.49, 14.825) -> (94.39, 14.825)
  line L3558 (97.4601, 15.4732) -> (97.2325, 15.1325)
  line L3559 (93.6475, 15.1325) -> (93.4199, 15.4732)
  line L3560 (93.4199, 15.4732) -> (93.34, 15.875)
  line L3561 (97.2325, 16.6175) -> (97.4601, 16.2768)
  line L3562 (94.39, 14.825) -> (93.9882, 14.9049)
  line L3563 (94.39, 16.925) -> (96.49, 16.925)
  line L3564 (96.49, 16.925) -> (96.8918, 16.8451)
  line L3565 (93.4199, 16.2768) -> (93.6475, 16.6175)
  line L3566 (93.6475, 16.6175) -> (93.9882, 16.8451)
  line L3567 (93.9882, 16.8451) -> (94.39, 16.925)
  line L3568 (97.54, 15.875) -> (97.4601, 15.4732)
  line L3569 (97.2325, 15.1325) -> (96.8918, 14.9049)
  line L3570 (96.8918, 16.8451) -> (97.2325, 16.6175)
  line L3571 (97.4601, 16.2768) -> (97.54, 15.875)
  line L3572 (21.2598, 76.1746) -> (20.9296, 76.5048)
  line L3573 (22.2504, 76.5048) -> (21.9202, 76.1746)
  line L3574 (21.9202, 77.4954) -> (22.2504, 77.1652)
  line L3575 (21.2598, 77.4954) -> (21.9202, 77.4954)
  line L3576 (21.9202, 76.1746) -> (21.2598, 76.1746)
  line L3577 (22.2504, 77.1652) -> (22.2504, 76.5048)
  line L3578 (20.9296, 77.1652) -> (21.2598, 77.4954)
  line L3579 (20.9296, 76.5048) -> (20.9296, 77.1652)
  line L3580 (24.4602, 76.1746) -> (23.7998, 76.1746)
  line L3581 (23.4696, 76.5048) -> (23.4696, 77.1652)
  line L3582 (23.7998, 76.1746) -> (23.4696, 76.5048)
  line L3583 (24.7904, 76.5048) -> (24.4602, 76.1746)
  line L3584 (23.4696, 77.1652) -> (23.7998, 77.4954)
  line L3585 (23.7998, 77.4954) -> (24.4602, 77.4954)
  line L3586 (24.7904, 77.1652) -> (24.7904, 76.5048)
  line L3587 (24.4602, 77.4954) -> (24.7904, 77.1652)
  line L3588 (79.0702, 76.8604) -> (79.4004, 76.5302)
  line L3589 (78.4098, 75.5396) -> (78.0796, 75.8698)
  line L3590 (78.0796, 75.8698) -> (78.0796, 76.5302)
  line L3591 (78.0796, 76.5302) -> (78.4098, 76.8604)
  line L3592 (79.4004, 75.8698) -> (79.0702, 75.5396)
  line L3593 (79.0702, 75.5396) -> (78.4098, 75.5396)
  line L3594 (78.4098, 76.8604) -> (79.0702, 76.8604)
  line L3595 (79.4004, 76.5302) -> (79.4004, 75.8698)
  line L3596 (76.8604, 75.8698) -> (76.5302, 75.5396)
  line L3597 (76.5302, 75.5396) -> (75.8698, 75.5396)
  line L3598 (75.5396, 75.8698) -> (75.5396, 76.5302)
  line L3599 (75.8698, 76.8604) -> (76.5302, 76.8604)
  line L3600 (76.5302, 76.8604) -> (76.8604, 76.5302)
  line L3601 (75.8698, 75.5396) -> (75.5396, 75.8698)
  line L3602 (75.5396, 76.5302) -> (75.8698, 76.8604)
  line L3603 (76.8604, 76.5302) -> (76.8604, 75.8698)
  line L3604 (10.8204, 16.1798) -> (10.4902, 15.8496)
  line L3605 (9.4996, 16.8402) -> (9.8298, 17.1704)
  line L3606 (10.4902, 17.1704) -> (10.8204, 16.8402)
  line L3607 (10.4902, 15.8496) -> (9.8298, 15.8496)
  line L3608 (10.8204, 16.8402) -> (10.8204, 16.1798)
  line L3609 (9.4996, 16.1798) -> (9.4996, 16.8402)
  line L3610 (9.8298, 17.1704) -> (10.4902, 17.1704)
  line L3611 (9.8298, 15.8496) -> (9.4996, 16.1798)
  line L3612 (12.3698, 17.1704) -> (13.0302, 17.1704)
  line L3613 (13.3604, 16.8402) -> (13.3604, 16.1798)
  line L3614 (13.0302, 15.8496) -> (12.3698, 15.8496)
  line L3615 (12.0396, 16.1798) -> (12.0396, 16.8402)
  line L3616 (12.3698, 15.8496) -> (12.0396, 16.1798)
  line L3617 (13.3604, 16.1798) -> (13.0302, 15.8496)
  line L3618 (13.0302, 17.1704) -> (13.3604, 16.8402)
  line L3619 (12.0396, 16.8402) -> (12.3698, 17.1704)
  line L3620 (79.4004, 16.1798) -> (79.0702, 15.8496)
  line L3621 (79.0702, 17.1704) -> (79.4004, 16.8402)
  line L3622 (78.4098, 17.1704) -> (79.0702, 17.1704)
  line L3623 (79.0702, 15.8496) -> (78.4098, 15.8496)
  line L3624 (78.4098, 15.8496) -> (78.0796, 16.1798)
  line L3625 (78.0796, 16.1798) -> (78.0796, 16.8402)
  line L3626 (78.0796, 16.8402) -> (78.4098, 17.1704)
  line L3627 (79.4004, 16.8402) -> (79.4004, 16.1798)
  line L3628 (75.8698, 15.8496) -> (75.5396, 16.1798)
  line L3629 (76.5302, 15.8496) -> (75.8698, 15.8496)
  line L3630 (76.5302, 17.1704) -> (76.8604, 16.8402)
  line L3631 (75.5396, 16.1798) -> (75.5396, 16.8402)
  line L3632 (75.8698, 17.1704) -> (76.5302, 17.1704)
  line L3633 (76.8604, 16.8402) -> (76.8604, 16.1798)
  line L3634 (75.5396, 16.8402) -> (75.8698, 17.1704)
  line L3635 (76.8604, 16.1798) -> (76.5302, 15.8496)
  line L3636 (67.6402, 15.8496) -> (66.9798, 15.8496)
  line L3637 (66.9798, 15.8496) -> (66.6496, 16.1798)
  line L3638 (66.6496, 16.1798) -> (66.6496, 16.8402)
  line L3639 (66.9798, 17.1704) -> (67.6402, 17.1704)
  line L3640 (67.6402, 17.1704) -> (67.9704, 16.8402)
  line L3641 (66.6496, 16.8402) -> (66.9798, 17.1704)
  line L3642 (67.9704, 16.1798) -> (67.6402, 15.8496)
  line L3643 (67.9704, 16.8402) -> (67.9704, 16.1798)
  line L3644 (64.4398, 17.1704) -> (65.1002, 17.1704)
  line L3645 (64.1096, 16.8402) -> (64.4398, 17.1704)
  line L3646 (65.1002, 17.1704) -> (65.4304, 16.8402)
  line L3647 (64.1096, 16.1798) -> (64.1096, 16.8402)
  line L3648 (65.4304, 16.8402) -> (65.4304, 16.1798)
  line L3649 (65.1002, 15.8496) -> (64.4398, 15.8496)
  line L3650 (65.4304, 16.1798) -> (65.1002, 15.8496)
  line L3651 (64.4398, 15.8496) -> (64.1096, 16.1798)
  line L3652 (56.8198, 15.8496) -> (56.4896, 16.1798)
  line L3653 (57.8104, 16.1798) -> (57.4802, 15.8496)
  line L3654 (57.4802, 15.8496) -> (56.8198, 15.8496)
  line L3655 (56.8198, 17.1704) -> (57.4802, 17.1704)
  line L3656 (56.4896, 16.1798) -> (56.4896, 16.8402)
  line L3657 (57.8104, 16.8402) -> (57.8104, 16.1798)
  line L3658 (57.4802, 17.1704) -> (57.8104, 16.8402)
  line L3659 (56.4896, 16.8402) -> (56.8198, 17.1704)
  line L3660 (54.9402, 17.1704) -> (55.2704, 16.8402)
  line L3661 (54.9402, 15.8496) -> (54.2798, 15.8496)
  line L3662 (54.2798, 17.1704) -> (54.9402, 17.1704)
  line L3663 (53.9496, 16.8402) -> (54.2798, 17.1704)
  line L3664 (53.9496, 16.1798) -> (53.9496, 16.8402)
  line L3665 (54.2798, 15.8496) -> (53.9496, 16.1798)
  line L3666 (55.2704, 16.1798) -> (54.9402, 15.8496)
  line L3667 (55.2704, 16.8402) -> (55.2704, 16.1798)
  line L3668 (45.6946, 16.8402) -> (46.0248, 17.1704)
  line L3669 (45.6946, 16.1798) -> (45.6946, 16.8402)
  line L3670 (46.6852, 17.1704) -> (47.0154, 16.8402)
  line L3671 (47.0154, 16.8402) -> (47.0154, 16.1798)
  line L3672 (46.6852, 15.8496) -> (46.0248, 15.8496)
  line L3673 (46.0248, 17.1704) -> (46.6852, 17.1704)
  line L3674 (47.0154, 16.1798) -> (46.6852, 15.8496)
  line L3675 (46.0248, 15.8496) -> (45.6946, 16.1798)
  line L3676 (48.2346, 16.8402) -> (48.5648, 17.1704)
  line L3677 (49.2252, 17.1704) -> (49.5554, 16.8402)
  line L3678 (49.5554, 16.8402) -> (49.5554, 16.1798)
  line L3679 (49.5554, 16.1798) -> (49.2252, 15.8496)
  line L3680 (48.5648, 17.1704) -> (49.2252, 17.1704)
  line L3681 (49.2252, 15.8496) -> (48.5648, 15.8496)
  line L3682 (48.5648, 15.8496) -> (48.2346, 16.1798)
  line L3683 (48.2346, 16.1798) -> (48.2346, 16.8402)
  line L3684 (36.2204, 16.1798) -> (35.8902, 15.8496)
  line L3685 (34.8996, 16.8402) -> (35.2298, 17.1704)
  line L3686 (36.2204, 16.8402) -> (36.2204, 16.1798)
  line L3687 (35.2298, 15.8496) -> (34.8996, 16.1798)
  line L3688 (35.8902, 15.8496) -> (35.2298, 15.8496)
  line L3689 (35.8902, 17.1704) -> (36.2204, 16.8402)
  line L3690 (35.2298, 17.1704) -> (35.8902, 17.1704)
  line L3691 (34.8996, 16.1798) -> (34.8996, 16.8402)
  line L3692 (38.7604, 16.8402) -> (38.7604, 16.1798)
  line L3693 (37.7698, 15.8496) -> (37.4396, 16.1798)
  line L3694 (38.4302, 17.1704) -> (38.7604, 16.8402)
  line L3695 (37.4396, 16.1798) -> (37.4396, 16.8402)
  line L3696 (37.7698, 17.1704) -> (38.4302, 17.1704)
  line L3697 (37.4396, 16.8402) -> (37.7698, 17.1704)
  line L3698 (38.7604, 16.1798) -> (38.4302, 15.8496)
  line L3699 (38.4302, 15.8496) -> (37.7698, 15.8496)
  line L3700 (22.1996, 16.8402) -> (22.5298, 17.1704)
  line L3701 (22.5298, 15.8496) -> (22.1996, 16.1798)
  line L3702 (23.5204, 16.8402) -> (23.5204, 16.1798)
  line L3703 (23.1902, 15.8496) -> (22.5298, 15.8496)
  line L3704 (22.1996, 16.1798) -> (22.1996, 16.8402)
  line L3705 (23.1902, 17.1704) -> (23.5204, 16.8402)
  line L3706 (22.5298, 17.1704) -> (23.1902, 17.1704)
  line L3707 (23.5204, 16.1798) -> (23.1902, 15.8496)
  line L3708 (26.0604, 16.1798) -> (25.7302, 15.8496)
  line L3709 (25.0698, 17.1704) -> (25.7302, 17.1704)
  line L3710 (24.7396, 16.8402) -> (25.0698, 17.1704)
  line L3711 (26.0604, 16.8402) -> (26.0604, 16.1798)
  line L3712 (25.7302, 15.8496) -> (25.0698, 15.8496)
  line L3713 (24.7396, 16.1798) -> (24.7396, 16.8402)
  line L3714 (25.7302, 17.1704) -> (26.0604, 16.8402)
  line L3715 (25.0698, 15.8496) -> (24.7396, 16.1798)
  line L3716 (90.8304, 16.8402) -> (90.8304, 16.1798)
  line L3717 (90.5002, 17.1704) -> (90.8304, 16.8402)
  line L3718 (90.8304, 16.1798) -> (90.5002, 15.8496)
  line L3719 (89.5096, 16.1798) -> (89.5096, 16.8402)
  line L3720 (89.8398, 15.8496) -> (89.5096, 16.1798)
  line L3721 (90.5002, 15.8496) -> (89.8398, 15.8496)
  line L3722 (89.8398, 17.1704) -> (90.5002, 17.1704)
  line L3723 (89.5096, 16.8402) -> (89.8398, 17.1704)
  line L3724 (88.2904, 16.1798) -> (87.9602, 15.8496)
  line L3725 (87.9602, 15.8496) -> (87.2998, 15.8496)
  line L3726 (86.9696, 16.8402) -> (87.2998, 17.1704)
  line L3727 (87.2998, 15.8496) -> (86.9696, 16.1798)
  line L3728 (86.9696, 16.1798) -> (86.9696, 16.8402)
  line L3729 (87.2998, 17.1704) -> (87.9602, 17.1704)
  line L3730 (88.2904, 16.8402) -> (88.2904, 16.1798)
  line L3731 (87.9602, 17.1704) -> (88.2904, 16.8402)
  line L3732 (18.3896, 76.5048) -> (18.3896, 77.1652)
  line L3733 (18.7198, 76.1746) -> (18.3896, 76.5048)
  line L3734 (18.7198, 77.4954) -> (19.3802, 77.4954)
  line L3735 (19.7104, 76.5048) -> (19.3802, 76.1746)
  line L3736 (19.3802, 77.4954) -> (19.7104, 77.1652)
  line L3737 (19.7104, 77.1652) -> (19.7104, 76.5048)
  line L3738 (18.3896, 77.1652) -> (18.7198, 77.4954)
  line L3739 (19.3802, 76.1746) -> (18.7198, 76.1746)
  line L3740 (8.5598, 77.4954) -> (9.2202, 77.4954)
  line L3741 (9.2202, 77.4954) -> (9.5504, 77.1652)
  line L3742 (8.2296, 76.5048) -> (8.2296, 77.1652)
  line L3743 (9.5504, 76.5048) -> (9.2202, 76.1746)
  line L3744 (9.5504, 77.1652) -> (9.5504, 76.5048)
  line L3745 (9.2202, 76.1746) -> (8.5598, 76.1746)
  line L3746 (8.5598, 76.1746) -> (8.2296, 76.5048)
  line L3747 (8.2296, 77.1652) -> (8.5598, 77.4954)
  line L3748 (80.9498, 75.5396) -> (80.6196, 75.8698)
  line L3749 (81.9404, 76.5302) -> (81.9404, 75.8698)
  line L3750 (80.6196, 76.5302) -> (80.9498, 76.8604)
  line L3751 (80.9498, 76.8604) -> (81.6102, 76.8604)
  line L3752 (81.6102, 75.5396) -> (80.9498, 75.5396)
  line L3753 (81.9404, 75.8698) -> (81.6102, 75.5396)
  line L3754 (81.6102, 76.8604) -> (81.9404, 76.5302)
  line L3755 (80.6196, 75.8698) -> (80.6196, 76.5302)
  line L3756 (92.1004, 75.8698) -> (91.7702, 75.5396)
  line L3757 (91.1098, 76.8604) -> (91.7702, 76.8604)
  line L3758 (91.7702, 76.8604) -> (92.1004, 76.5302)
  line L3759 (90.7796, 75.8698) -> (90.7796, 76.5302)
  line L3760 (92.1004, 76.5302) -> (92.1004, 75.8698)
  line L3761 (91.7702, 75.5396) -> (91.1098, 75.5396)
  line L3762 (91.1098, 75.5396) -> (90.7796, 75.8698)
  line L3763 (90.7796, 76.5302) -> (91.1098, 76.8604)
  line L3764 (10.4902, 19.6596) -> (9.8298, 19.6596)
  line L3765 (9.8298, 20.9804) -> (10.4902, 20.9804)
  line L3766 (9.8298, 19.6596) -> (9.4996, 19.9898)
  line L3767 (10.8204, 19.9898) -> (10.4902, 19.6596)
  line L3768 (9.4996, 19.9898) -> (9.4996, 20.6502)
  line L3769 (10.8204, 20.6502) -> (10.8204, 19.9898)
  line L3770 (9.4996, 20.6502) -> (9.8298, 20.9804)
  line L3771 (10.4902, 20.9804) -> (10.8204, 20.6502)
  line L3772 (9.4996, 30.1498) -> (9.4996, 30.8102)
  line L3773 (9.4996, 30.8102) -> (9.8298, 31.1404)
  line L3774 (10.8204, 30.1498) -> (10.4902, 29.8196)
  line L3775 (10.4902, 31.1404) -> (10.8204, 30.8102)
  line L3776 (9.8298, 29.8196) -> (9.4996, 30.1498)
  line L3777 (9.8298, 31.1404) -> (10.4902, 31.1404)
  line L3778 (10.4902, 29.8196) -> (9.8298, 29.8196)
  line L3779 (10.8204, 30.8102) -> (10.8204, 30.1498)
  line L3780 (23.1902, 20.9804) -> (23.5204, 20.6502)
  line L3781 (22.5298, 19.6596) -> (22.1996, 19.9898)
  line L3782 (22.1996, 20.6502) -> (22.5298, 20.9804)
  line L3783 (22.1996, 19.9898) -> (22.1996, 20.6502)
  line L3784 (23.1902, 19.6596) -> (22.5298, 19.6596)
  line L3785 (22.5298, 20.9804) -> (23.1902, 20.9804)
  line L3786 (23.5204, 19.9898) -> (23.1902, 19.6596)
  line L3787 (23.5204, 20.6502) -> (23.5204, 19.9898)
  line L3788 (23.1902, 29.8196) -> (22.5298, 29.8196)
  line L3789 (23.5204, 30.1498) -> (23.1902, 29.8196)
  line L3790 (22.5298, 29.8196) -> (22.1996, 30.1498)
  line L3791 (23.1902, 31.1404) -> (23.5204, 30.8102)
  line L3792 (22.1996, 30.1498) -> (22.1996, 30.8102)
  line L3793 (22.1996, 30.8102) -> (22.5298, 31.1404)
  line L3794 (23.5204, 30.8102) -> (23.5204, 30.1498)
  line L3795 (22.5298, 31.1404) -> (23.1902, 31.1404)
  line L3796 (34.8996, 19.9898) -> (34.8996, 20.6502)
  line L3797 (34.8996, 20.6502) -> (35.2298, 20.9804)
  line L3798 (35.8902, 20.9804) -> (36.2204, 20.6502)
  line L3799 (35.2298, 19.6596) -> (34.8996, 19.9898)
  line L3800 (36.2204, 20.6502) -> (36.2204, 19.9898)
  line L3801 (36.2204, 19.9898) -> (35.8902, 19.6596)
  line L3802 (35.8902, 19.6596) -> (35.2298, 19.6596)
  line L3803 (35.2298, 20.9804) -> (35.8902, 20.9804)
  line L3804 (35.2298, 31.1404) -> (35.8902, 31.1404)
  line L3805 (36.2204, 30.1498) -> (35.8902, 29.8196)
  line L3806 (34.8996, 30.1498) -> (34.8996, 30.8102)
  line L3807 (35.8902, 31.1404) -> (36.2204, 30.8102)
  line L3808 (35.2298, 29.8196) -> (34.8996, 30.1498)
  line L3809 (35.8902, 29.8196) -> (35.2298, 29.8196)
  line L3810 (36.2204, 30.8102) -> (36.2204, 30.1498)
  line L3811 (34.8996, 30.8102) -> (35.2298, 31.1404)
  line L3812 (48.9204, 20.6502) -> (48.9204, 19.9898)
  line L3813 (48.9204, 19.9898) -> (48.5902, 19.6596)
  line L3814 (47.9298, 19.6596) -> (47.5996, 19.9898)
  line L3815 (47.9298, 20.9804) -> (48.5902, 20.9804)
  line L3816 (47.5996, 20.6502) -> (47.9298, 20.9804)
  line L3817 (48.5902, 19.6596) -> (47.9298, 19.6596)
  line L3818 (47.5996, 19.9898) -> (47.5996, 20.6502)
  line L3819 (48.5902, 20.9804) -> (48.9204, 20.6502)
  line L3820 (47.5996, 30.1498) -> (47.5996, 30.8102)
  line L3821 (47.5996, 30.8102) -> (47.9298, 31.1404)